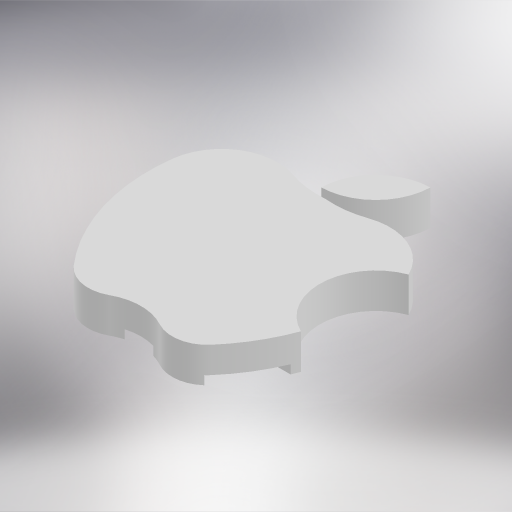
# Autodesk Inventor part: Apple_logo_white
Saved by Autodesk Inventor 2024 (Build 280153000, 153)
## iProperties
Created: 2023-10-30
Part Number: Apple_logo_white
Material: Generic
Document SubType Name: Modeling
Designer: SSAFY
Density: 1 g/cm^3
Appearance: Default
Author: SSAFY
Autodesk Inventor part; units mm, degrees
ref_plane "YZ Plane" through (0, 0, 0) normal (1, 0, 0) x (0, 1, 0)
ref_plane "XZ Plane" through (0, 0, 0) normal (0, 1, 0) x (-1, 0, 0)
ref_plane "XY Plane" through (0, 0, 0) normal (0, 0, 1) x (1, 0, 0)
sketch "Sketch2" plane through (0, 0, 0) normal (0, 1, 0) x (-1, 0, 0)
  line L0 (0, 0) -> (-15.3807, 0) construction
  line L1 (0, 12) -> (0, -86.6461) construction
  circle A0 centre (0, 0) radius 2
  circle A1 centre (-12, 0) radius 10
  circle A2 centre (-23.3137, -11.3137) radius 6
  circle A3 centre (-16, -32.0624) radius 16
  line L2 (-16, -48.0624) -> (0, -48.0624)
  line L3 (-12, 10) -> (0, 10)
  line L4 (-12, 0) -> (-23.3137, -11.3137)
  arc A4 (-19.5628, 6.5425) -> (-31.8772, -34.041) centre (19.8923, -27.5896) ccw
  line L5 (0, 0) -> (15.3807, 0) construction
  circle A5 centre (0, 0) radius 2
  circle A6 centre (12, 0) radius 10
  circle A7 centre (23.3137, -11.3137) radius 6
  circle A8 centre (16, -32.0624) radius 16
  line L6 (16, -48.0624) -> (0, -48.0624)
  line L7 (12, 10) -> (0, 10)
  line L8 (12, 0) -> (23.3137, -11.3137)
  arc A9 (31.8772, -34.041) -> (19.5628, 6.5425) centre (-19.8923, -27.5896) ccw
  arc A10 (10.7519, -47.1773) -> (0, -45.8341) centre (2.2238, -71.7388) ccw
  arc A11 (0, 6.9317) -> (7.2, 8.7727) centre (0, 21.9317) ccw
  arc A12 (0, -45.8341) -> (-10.7519, -47.1773) centre (-2.2238, -71.7388) ccw
  arc A13 (-7.2, 8.7727) -> (0, 6.9317) centre (0, 21.9317) ccw
  line L9 (-23.3137, -11.3137) -> (-58.3661, -46.3661)
  line L10 (-12, 0) -> (-38.3514, 26.3514)
  line L11 (10.1546, -70.2379) -> (-38.6751, -21.4081)
  circle A14 centre (-36.0416, -24.0416) radius 16
  circle A15 centre (-12.4253, -47.658) radius 16
  circle A16 centre (3.9792, -64.0624) radius 16
  point P0 (3.5695, -48.0677)
  point P1 (-12.0156, -63.6527)
  point P2 (-7.2, 8.7727)
  point P3 (-29.0893, -9.6311)
  point P4 (-30.4093, -39.0175)
  point P5 (-10.7519, -47.1773)
  dimension "d0" = 4
  dimension "d1" = 20
  dimension "d2" = 12
  dimension "d3" = 32
  dimension "d4" = 135
  dimension "d6" = 26
  dimension "d7" = 15
  dimension "d8" = 90
  dimension "d12" = 34
  dimension "d13" = 32
  dimension "d14" = 32
  dimension "d15" = 32
  constraints: 24 end point, 24 point on circle, 17 centre point, 13 symmetric about line, 13 tangent, 11 point on line, 2 coincident, 2 horizontal, 1 collinear, 1 parallel, 1 vertical, 7 other
  measures "d0" diameter of A0
  measures "d1" diameter of A1
  measures "d2" diameter of A2
  measures "d3" diameter of A3
  measures "d4" angle of L4 L0
  measures "d6" radius of A10
  measures "d7" radius of A11
  measures "d8" angle of L10 L4
  measures "d12" distance between parallel lines of L10 L11
  measures "d13" diameter of A14
  measures "d14" diameter of A15
  measures "d15" diameter of A16
extrude "Extrusion1" add sketch "Sketch2" along normal blind 10 contours A0 | A6 A7 A8 A3 A2 A1 A0 | A0 A1 A13 A11 A6 | A6 | A1 L4 L10 | A6 A9 A7 | A7 | A2 A4 A1 | L4 L9 A14 A2 | A1 L10 L4 | A2 A14 L9 L4 | A9 A8 A7 | A8 | A2 A14 A4 | A3 A15 L11 A14 | A8 A10 A15 A3 | A3 A14 A2 | A15 A10 A12 A3 | A3 L11 A15 | A15 A3 A14 L11 | L11 A3 A15 | A15 L11 A16 | A16 L11 A15
sketch "Sketch3" plane through (0, 0, 0) normal (0, -1, 0) x (1, 0, 0)
  arc A0 (19.5628, 6.5425) -> (7.2, 8.7727) centre (12, 0) ccw construction
  line L0 (-55.1507, 7.5) -> (56.5925, 7.5)
  line L1 (56.5925, 7.5) -> (56.5925, -7.5)
  line L2 (56.5925, -7.5) -> (-55.1507, -7.5)
  line L3 (-55.1507, -7.5) -> (-55.1507, 7.5)
  point P0 (0, 0)
  dimension "d18" = 15
  dimension "d19" = 7.5
  constraints: 8 end point, 2 parallel, 1 horizontal, 1 perpendicular
  measures "d18" distance of L0.end L1.end
  measures "d19" distance from line of A0.centre L0
extrude "Extrusion2" cut sketch "Sketch3" against normal blind 2.5
equation "\"d19\" = 0.5 * d18"
body "Solid1"
